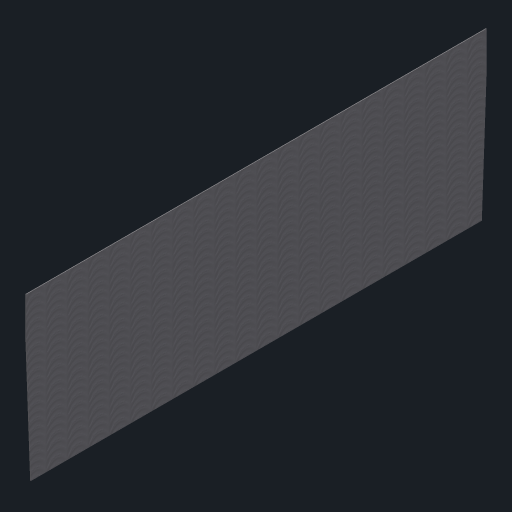
# Autodesk Inventor part: CHAPA_2
Saved by Autodesk Inventor 2024.3 (Build 283343000, 343)
## iProperties
Created: 2024-06-14
Part Number: CHAPA_2
Material: Steel, Mild, Welded
Document SubType Name: Sheet Metal
Designer: Niler
Density: 7.85 g/cm^3
Sheet Metal Rule: Default
Appearance: Weld - Steel Mild
Author: Niler
Autodesk Inventor part; units mm, degrees
ref_plane "YZ Plane" through (0, 0, 0) normal (1, 0, 0) x (0, 1, 0)
ref_plane "XZ Plane" through (0, 0, 0) normal (0, 1, 0) x (-1, 0, 0)
ref_plane "XY Plane" through (0, 0, 0) normal (0, 0, 1) x (1, 0, 0)
sketch "Sketch1" plane through (0, 0, 0) normal (1, 0, 0) x (0, 1, 0)
  line L0 (-41.95, 491.5) -> (41.95, 491.5)
  line L1 (41.95, 491.5) -> (41.95, -491.5)
  line L2 (41.95, -491.5) -> (-41.95, -491.5)
  line L3 (-41.95, -491.5) -> (-41.95, 491.5)
  line L4 (-41.95, 491.5) -> (41.95, -491.5) construction
  line L5 (41.95, 491.5) -> (-41.95, -491.5) construction
  line L6 (-41.95, 491.5) -> (-988.2655, 455.5)
  line L7 (-988.2655, 455.5) -> (-988.2655, -455.5)
  line L8 (-988.2655, -455.5) -> (-41.95, -491.5)
  line L9 (-308.05, 481.3769) -> (-308.05, -481.3769)
  point P0 (0, 0)
  point P1 (-988.2655, 0)
  point P2 (-41.95, 0)
  dimension "d0" = 983
  dimension "d1" = 83.9
  dimension "d3" = 911
  dimension "d4" = 947
  dimension "d5" = 350
  measures "d0" distance of L0.end L1.end
  measures "d1" distance of L0.start L0.end
  measures "d3" distance of L6.end L7.end
  measures "d4" distance of L0.start L6.end
  measures "d5" distance between parallel lines of L9 L1
extrude "Plate1" add sketch "Sketch1" along normal blind 1.5 contours L0 L1 L2 L3 | L3 L8 L9 L6
equation "\"d6\" = Thickness"
equation "\"BendRadius\" = Thickness"
equation "\"BendReliefWidth\" = Thickness"
equation "\"BendReliefDepth\" = 0.5 * Thickness"
equation "\"CornerReliefSize\" = 4 * Thickness"
equation "\"MinimumRemnant\" = 2 * Thickness"
equation "\"TransitionRadius\" = BendRadius"
equation "\"JacobiRadiusSize\" = BendRadius"
equation "\"GapSize\" = Thickness"
equation "\"Thickness\" = 1.5"
body "Solid1"
